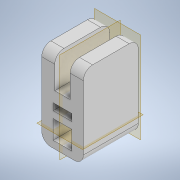
# Autodesk Inventor part: fuselage_honeycomb_interface_v2
Saved by Autodesk Inventor 2021 (Build 250183000, 183)
## iProperties
Created: 2020-12-06
Part Number: fuselage_honeycomb_interface_v2
Material: Generic
Document SubType Name: Modeling
Designer: victo
Density: 1 g/cm^3
Appearance: Default
Mass: 1.37955 g
Surface Area: 13.451 cm^2
Volume: 1.37955 cm^3
Author: victo
Autodesk Inventor part; units mm, degrees
sketch "Sketch1" plane through (0, 0, 0) normal (0, 0, 1) x (1, 0, 0)
  line L0 (-4.55, 7.5) -> (4.55, 7.5)
  line L1 (4.55, 7.5) -> (4.55, -7.5)
  line L2 (4.55, -7.5) -> (-4.55, -7.5)
  line L3 (-4.55, -7.5) -> (-4.55, 7.5)
  line L4 (-4.55, 7.5) -> (4.55, -7.5) construction
  line L5 (4.55, 7.5) -> (-4.55, -7.5) construction
  line L6 (-2.05, -2.05) -> (2.05, -2.05)
  line L7 (2.05, -2.05) -> (2.05, 2.05)
  line L8 (2.05, 2.05) -> (-2.05, 2.05)
  line L9 (-2.05, 2.05) -> (-2.05, -2.05)
  line L10 (-2.05, -2.05) -> (2.05, 2.05) construction
  line L11 (2.05, -2.05) -> (-2.05, 2.05) construction
  line L12 (-4.55, 6) -> (-4.55, 7.5)
  line L13 (-4.55, -6) -> (-4.55, -7.5)
  line L14 (4.55, 6) -> (4.55, 7.5)
  line L15 (4.55, -6) -> (4.55, -7.5)
  point P0 (0, 0)
  point P1 (16.55, 6)
  dimension "d1" = 9.1
  dimension "d2" = 4.1
  dimension "d3" = 4.1
  constraints: 32 end point, 4 midpoint, 4 parallel, 2 horizontal, 2 perpendicular
  measures "d1" distance of L0.start L0.end
  measures "d2" distance of L7.end L8.end
  measures "d3" distance of L6.end L7.end
extrude "Extrusion1" add sketch "Sketch1" along normal blind 12
sketch "Sketch2" plane through (0, 0, 12) normal (0, 0, 1) x (1, 0, 0)
  line L0 (4.55, 7.5) -> (-4.55, 7.5) projected
  line L1 (-4.55, 7.5) -> (-1.7, 7.5)
  line L2 (-1.7, 7.5) -> (-1.7, 14.5)
  line L3 (-1.7, 14.5) -> (-4.55, 14.5)
  line L4 (-4.55, 14.5) -> (-4.55, 7.5)
  line L5 (1.7, 7.5) -> (4.55, 7.5)
  line L6 (4.55, 7.5) -> (4.55, 14.5)
  line L7 (4.55, 14.5) -> (1.7, 14.5)
  line L8 (1.7, 14.5) -> (1.7, 7.5)
  point P0 (0, 0)
  point P1 (16.55, 7.5)
  point P2 (-16.55, 7.5)
  dimension "d15" = 2.85
  dimension "d16" = 2.85
  dimension "d17" = 7
  dimension "d18" = 7
  dimension "d19" = 1.7
  dimension "d20" = 1.7
  constraints: 16 end point, 4 parallel, 2 horizontal, 2 perpendicular, 2 point on line
  measures "d15" distance of L6.end L7.end
  measures "d16" distance of L2.end L3.end
  measures "d17" distance of L1.end L2.end
  measures "d18" distance of L5.end L6.end
  measures "d19" distance from line of point (0, 0) L8
  measures "d20" distance from line of point (0, 0) L2
extrude "Extrusion2" add sketch "Sketch2" against normal up to surface (12 mm away)
sketch "Sketch5" plane through (0, 0, 0) normal (0, 0, -1) x (-1, 0, 0)
  line L0 (-2.05, 5.05) -> (2.05, 5.05)
  line L1 (2.05, 5.05) -> (2.05, 3.55)
  line L2 (2.05, 3.55) -> (-2.05, 3.55)
  line L3 (-2.05, 3.55) -> (-2.05, 5.05)
  line L4 (-2.05, -3.55) -> (2.05, -3.55)
  line L5 (2.05, -3.55) -> (2.05, -5.05)
  line L6 (2.05, -5.05) -> (-2.05, -5.05)
  line L7 (-2.05, -5.05) -> (-2.05, -3.55)
  line L8 (2.05, 2.05) -> (-2.05, 2.05) projected
  line L9 (2.05, -2.05) -> (2.05, 2.05) projected
  line L10 (-2.05, -2.05) -> (2.05, -2.05) projected
  point P0 (0, 0)
  dimension "d31" = 4.1
  dimension "d32" = 4.1
  dimension "d33" = 1.5
  dimension "d34" = 1.5
  dimension "d35" = 1.5
  dimension "d36" = 1.5
  constraints: 16 end point, 4 parallel, 2 horizontal, 2 perpendicular, 2 point on line, 1 collinear
  measures "d31" distance of L0.start L0.end
  measures "d32" distance of L8.start L8.end
  measures "d33" distance between parallel lines of L8 L2
  measures "d34" distance of L0.end L1.end
  measures "d35" distance between parallel lines of L4 L10
  measures "d36" distance of L4.end L5.end
extrude "Extrusion4" cut sketch "Sketch5" against normal through all
sketch "Sketch6" plane through (0, 0, 12) normal (0, 0, 1) x (1, 0, 0)
  line L0 (-4.55, 14.5) -> (-4.55, -7.5) projected
  line L1 (-4.55, -7.5) -> (4.55, -7.5) projected
  line L2 (-4.55, -3.55) -> (4.55, -3.55)
  line L3 (4.55, -3.55) -> (4.55, -7.5)
  line L4 (4.55, -7.5) -> (-4.55, -7.5)
  line L5 (-4.55, -7.5) -> (-4.55, -3.55)
  line L6 (-2.05, -3.55) -> (2.05, -3.55) projected
  point P0 (0, 0)
  dimension "d42" = 0
  constraints: 8 end point, 2 parallel, 1 horizontal, 1 perpendicular, 1 point on line
  measures "d42" distance between parallel lines of L6 L2
extrude "Extrusion5" cut sketch "Sketch6" against normal through all
fillet "Fillet3" radius 2 6 edges at (4.55, -3.55, 6) (-4.55, -3.55, 6) (3.125, 14.5, 12) (-3.125, 14.5, 12) (-3.125, 14.5, 0) (3.125, 14.5, 0)
equation "\"d31\" = d32"
body "Solid1"
